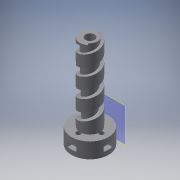
# Autodesk Inventor part: screwServoBlock
Saved by Autodesk Inventor 2017 (Build 210142000, 142)
## iProperties
Created: 2016-10-16
Part Number: screwServoBlock
Material: Generic
Document SubType Name: Modeling
Designer: Bardo91
Density: 1 g/cm^3
Appearance: Default
Author: Bardo91
Autodesk Inventor part; units mm, degrees
ref_plane "YZ Plane" through (0, 0, 0) normal (1, 0, 0) x (0, 1, 0)
ref_plane "XY Plane" through (0, 0, 0) normal (0, 0, 1) x (1, 0, 0)
sketch "Sketch1" plane through (0, 0, 0) normal (0, 0, 1) x (1, 0, 0)
  line L0 (0, 0) -> (0, 7.5)
  circle A0 centre (0, 7.5) radius 1.5
  circle A1 centre (-5.3033, 5.3033) radius 1.5
  circle A2 centre (-7.5, 0) radius 1.5
  circle A3 centre (-5.3033, -5.3033) radius 1.5
  circle A4 centre (0, -7.5) radius 1.5
  circle A5 centre (5.3033, -5.3033) radius 1.5
  circle A6 centre (7.5, 0) radius 1.5
  circle A7 centre (5.3033, 5.3033) radius 1.5
  circle A8 centre (0, 0) radius 12
  dimension "d0" = 7.5
  dimension "d1" = 3
  dimension "d4" = 360
  dimension "d6" = 24
  constraints: 9 centre point, 2 coincident, 2 end point, 1 vertical, 17 other
  measures "d0" distance of L0.start L0.end
  measures "d1" diameter of A0
  measures "d6" diameter of A8
extrude "Extrusion1" add sketch "Sketch1" along normal blind 10 contours A1 | A3 | A5 | A7 | A8
sketch "Sketch2" plane through (0, 0, 0) normal (0, 0, -1) x (-1, 0, 0)
  circle A0 centre (0, 0) radius 6.5
  dimension "d9" = 13
  constraints: 1 centre point, 1 coincident
  measures "d9" diameter of A0
extrude "Extrusion2" cut sketch "Sketch2" against normal blind 1
sketch "Sketch3" plane through (0, 0, 10) normal (0, 0, 1) x (1, 0, 0)
  circle A0 centre (0, 0) radius 6.5
  dimension "d12" = 13
  constraints: 1 centre point, 1 coincident
  measures "d12" diameter of A0
extrude "Extrusion3" add sketch "Sketch3" along normal blind 50
sketch "Sketch5" plane through (0, 0, 60) normal (0, 0, 1) x (1, 0, 0)
  circle A0 centre (0, 0) radius 3
  dimension "d25" = 6
  constraints: 1 centre point, 1 coincident
  measures "d25" diameter of A0
extrude "Extrusion5" cut sketch "Sketch5" against normal up to surface (59 mm away)
ref_plane "Work Plane1" through (0, 12, 0) normal (0, 1, 0) x (-1, 0, 0)
sketch "Sketch7" plane through (0, 12, 0) normal (0, 1, 0) x (-1, 0, 0)
  line L0 (0, 0) -> (0, 3)
  line L1 (0, 3) -> (2.75, 3)
  line L2 (2.75, 3) -> (2.75, 6)
  line L3 (2.75, 6) -> (-2.75, 6)
  line L4 (-2.75, 6) -> (-2.75, 3)
  line L5 (-2.75, 3) -> (0, 3)
  dimension "d35" = 3
  dimension "d36" = 2.75
  dimension "d37" = 3
  dimension "d38" = 5.5
  constraints: 12 end point, 4 perpendicular, 1 horizontal, 1 vertical
  measures "d35" distance of L0.start L0.end
  measures "d36" distance of L0.end L1.end
  measures "d37" distance of L1.end L2.end
  measures "d38" distance of L2.end L3.end
extrude "Extrusion7" cut sketch "Sketch7" against normal blind 8
pattern_circular "Circular Pattern1" count 4 over 360 about axis through (0, 0, 60) along (0, 0, -1) of "Extrusion7"
sketch "Sketch8" plane through (0, 0, 10) normal (0, 0, 1) x (1, 0, 0)
  circle A0 centre (0, 0) radius 3
  dimension "d44" = 6
  constraints: 1 centre point, 1 coincident
  measures "d44" diameter of A0
extrude "Extrusion8" cut sketch "Sketch8" against normal through all
sketch "Sketch9" plane through (0, 0, 0) normal (1, 0, 0) x (0, 1, 0)
  line L0 (6.5, 10) -> (6.5, 60) projected
  line L1 (6.5, 10) -> (6.5, 60) projected
  line L2 (6.4167, 10) -> (9, 10) projected
  line L3 (9, 10) -> (4, 10)
  line L4 (4, 10) -> (4, 15)
  line L5 (4, 15) -> (9, 15)
  line L6 (9, 15) -> (9, 10)
  point P0 (0, 0)
  dimension "d61" = 5
  dimension "d62" = 5
  constraints: 8 end point, 2 parallel, 1 horizontal, 1 perpendicular
  measures "d61" distance of L4.end L5.end
  measures "d62" distance of L3.end L4.end
coil "Coil2" sketch "Sketch9" operation cut axis through (0, 0, 10) along (0, 0, 1) pitch 12.5 turns 4 hand right taper 1
body "Solid1"
